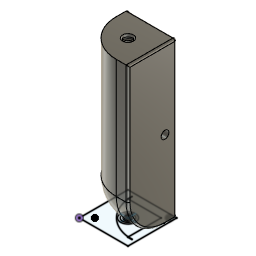
casestand (Autodesk Fusion 360 design; units mm, degrees)
Autodesk Fusion 360 part; units mm, degrees
sketch "main" plane through (0, 0, 0) normal (0, 0, 1) x (1, 0, 0)
  line L0 (0, 0) -> (25, 0)
  line L1 (25, 0) -> (25, 25)
  line L2 (25, 25) -> (0, 25)
  line L3 (0, 25) -> (0, 0)
  circle A0 centre (12.5, 12.5) radius 2.8
  circle A1 centre (12.5, 12.5) radius 3.8
  line L4 (8.7, 12.5) -> (16.3, 12.5)
  line L5 (12.5, 16.3) -> (12.5, 8.7)
  line L6 (4, 21) -> (21, 21)
  line L7 (21, 21) -> (21, 4)
  line L8 (21, 4) -> (23, 4)
  line L9 (4, 23) -> (4, 21)
  arc A2 (4, 23) -> (23, 4) centre (23, 23) ccw
  circle A3 centre (12.5, 12.5) radius 1.75
  point P0 (4, 4)
  dimension "d3" = 25
  dimension "d4" = 25
  dimension "d13" = 5.6
  dimension "d14" = 12.5
  dimension "d15" = 12.5
  dimension "d20" = 7.6
  dimension "d28" = 17
  dimension "d29" = 17
  dimension "d30" = 4
  dimension "d31" = 4
  dimension "d32" = 19
  dimension "d37" = 3.5
  constraint horizontal L0
  constraint vertical L1
  constraint horizontal L2
  constraint vertical L3
  constraint coincident L0.start L3.end
  constraint concentric A0 A1
  constraint coincident A1 L4.start
  constraint coincident A1 L4.end
  constraint parallel L2 L4
  constraint coincident A1 L5.start
  constraint coincident A1 L5.end
  constraint perpendicular L4 L5
  constraint horizontal L6
  constraint vertical L7
  constraint horizontal L8
  constraint vertical L9
  constraint coincident P0 L8
  constraint coincident P0 L9
  constraint tangent L8 A2
  constraint tangent L9 A2
  constraint concentric A1 A3
  measures "d3" distance of L0.start L0.end
  measures "d4" distance of L0.start L2.end
  measures "d13" diameter of A0
  measures "d14" distance of L0 A0.centre
  measures "d15" distance of L3 A0.centre
  measures "d20" diameter of A1
  measures "d28" distance of L6.start L6.end
  measures "d29" distance of L6.start P0
  measures "d30" distance of L0 L8
  measures "d31" distance of L3 L9
  measures "d32" radius of A2
  measures "d37" diameter of A3
extrude "Extrude1" add sketch "main" along normal blind 80 contours L0 L1 L2 L3 | A0 L4 L5 A3 | A0 A1 L4 L5 | A0 L4 L5 A3 | A0 A1 L4 L5 | A0 L4 L5 A3 | A0 A1 L4 L5 | A0 A1 L4 L5 | A0 L4 L5 A3 | L4 L5 A3 | L4 L5 A3 | L4 L5 A3 | L4 L5 A3 | L6 L9 A2 | L7 L8 A2 | L6 L7 A2
extrude "Extrude6" cut sketch "main" against normal blind 16 from surface at 80 contours L4 L5 A3 | L4 L5 A3 | L4 L5 A3 | L4 L5 A3
extrude "Extrude2" cut sketch "main" against normal blind 6 from surface at 80 contours A0 L4 L5 A3 | A0 L4 L5 A3 | A0 L4 L5 A3 | A0 L4 L5 A3 | L4 L5 A3 | L4 L5 A3 | L4 L5 A3 | L4 L5 A3
fillet "Fillet1" radius 19 2 edges at (0, 12.5, 0) (12.5, 0, 0)
fillet "Fillet2" radius 19 2 edges at (5.565, 5.565, 5.565) (0, 0, 49.5)
fillet "Fillet3" radius 1 9 edges at (25, 22, 0) (25, 5.565, 5.565) (25, 0, 49.5) (25, 25, 40) (22, 25, 0) (5.565, 25, 5.565) (0, 25, 49.5) (25, 12.5, 80) (12.5, 25, 80)
extrude "Extrude5" cut sketch "main" along normal up to surface (55 mm away) from surface at 15 contours A0 L4 L5 A3 | A0 A1 L4 L5 | A0 L4 L5 A3 | A0 A1 L4 L5 | A0 L4 L5 A3 | A0 A1 L4 L5 | A0 A1 L4 L5 | A0 L4 L5 A3 | L4 L5 A3 | L4 L5 A3 | L4 L5 A3 | L4 L5 A3 | L6 L7 A2
extrude "Extrude3" cut sketch "main" against normal blind 1.5 from surface at 78.5 contours A0 A1 L4 L5 | A0 A1 L4 L5 picked at (15.9538, 12.3197) picked at (9.0557, 12.8131)
extrude "Extrude4" cut sketch "main" along normal blind 1.5 from surface at 74 contours A0 A1 L4 L5 | A0 A1 L4 L5 picked at (12.8131, 15.9443) picked at (12.3197, 9.0462)
sketch "Sketch2" plane through (25, 0, 0) normal (1, 0, 0) x (0, 1, 0)
  line L0 (1, 79) -> (1, 19)
  arc A0 (1, 19) -> (19, 1) centre (19, 19) ccw
  line L1 (19, 1) -> (24, 1)
  line L2 (24, 1) -> (24, 79)
  line L3 (24, 79) -> (1, 79)
  circle A1 centre (19, 40) radius 2
  line L4 (25, 1) -> (25, 79)
  line L5 (24, 80) -> (0, 80)
  dimension "d43" = 4
  dimension "d47" = 6
  dimension "d48" = 40
  measures "d43" diameter of A1
  measures "d47" distance of A1.centre L4
  measures "d48" distance of A1.centre L5
extrude "Extrude7" cut sketch "Sketch2" against normal blind 10 contours A1
equation "width = 25 mm"
equation "height = 80 mm"
equation "d3 = width"
equation "d4 = width"
equation "d5 = height"
equation "r_side = 19 mm"
equation "r_bottom = 19 mm"
equation "d9 = r_bottom"
equation "d10 = r_side"
equation "hole_l = 6 mm"
equation "hole_d = 5.6 mm"
equation "d13 = hole_d"
equation "d14 = width / 2"
equation "d15 = width / 2"
equation "d17 = -hole_l"
equation "d20 = hole_d + 2 mm"
equation "d21 = -hole_l / 4"
equation "d24 = -hole_l"
equation "wall = 4 mm"
equation "d28 = width - 2 * wall"
equation "d29 = width - 2 * wall"
equation "d30 = wall"
equation "d31 = wall"
equation "d32 = r_side"
equation "d33 = r_bottom - wall"
equation "d34 = -wall - hole_l"
equation "screw_d = 3.5 mm"
equation "d37 = screw_d"
equation "d39 = -10 mm - hole_l"
equation "d47 = wall + 2 mm"
equation "d48 = height / 2"
named bodies: "casestand"
